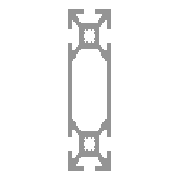
# Autodesk Inventor part: 3 842 992 992-2mm
Saved by Autodesk Inventor 2011 SP1 (Build 150282100, 282)
## iProperties
Created: 2011-02-10
Part Number: 3 842 992 992-2mm
Document SubType Name: Modeling
Designer: S. Wile
Density: 2.71 g/cm^3
Categories: <MemberInstance><Categories><Category DisplayName="Structural Shapes" InternalName="089c4875-fa83-4c05-b084-43b9cc11f5ed" Mnemonic="GRDR"><CategoryParameter DisplayName="Custom Base Point" InternalName="4f1d1b73-316d-484b-a3df-9cbabb16eb77" Mnemonic="shpBasePoint"/><CategoryParameter DisplayName="FG Authored" InternalName="9c666724-f362-4ea7-ac62-f6a007de5c69" Mnemonic="shpFGAuto"/><CategoryParameter DisplayName="Legacy Member ID" InternalName="340afe4f-75d7-48d3-ab7d-943f3c3da468" Mnemonic="LegacyMemberID"/><CategoryParameter DisplayName="Base Length" InternalName="42e34263-8f20-4d0e-ad48-bf1385b87c24" Mnemonic="shplen"/><CategoryParameter DisplayName="Distance of the Center of Gravity X-X" InternalName="26c9bdb8-9c79-4b4f-a92e-8e197583c9c4" Mnemonic="grcendistX"/><CategoryParameter DisplayName="Distance of the Center of Gravity Y-Y" InternalName="bcc4fb17-7af4-436a-8f8c-d0aa3b0248c5" Mnemonic="grcendistY"/><CategoryParameter DisplayName="Torsional Rigidity Modulus" InternalName="26c1ec35-5026-4c63-ad0a-751cf684a536" Mnemonic="torrigmod"/><CategoryParameter DisplayName="Torsional Section Modulus" InternalName="7c55a8dc-8844-49f9-a867-cc677b30ec9a" Mnemonic="torsecmod"/><CategoryParameter DisplayName="Coefficient of Shear Displacement" InternalName="de4c90c6-aaa8-468f-a335-6737b311b5d3" Mnemonic="shdispc"/><CategoryParameter DisplayName="Section Area" InternalName="1ff91680-64b0-4202-b9a3-7fd3f94bba3b" Mnemonic="secarea"/><CategoryParameter DisplayName="Moment of Inertia (x)" InternalName="4cd780bc-73d7-43ac-917a-579e5cbd684d" Mnemonic="inermomx"/><CategoryParameter DisplayName="Moment of Inertia (y)" InternalName="4b9f58ea-bced-460e-81ea-3d29ca5a49e3" Mnemonic="inermomy"/><CategoryParameter DisplayName="Section Module (x)" InternalName="72cfad18-cf51-4ed4-aaa7-c6b224f8419f" Mnemonic="secmodx"/><CategoryParameter DisplayName="Section Module (y)" InternalName="59eaa5e9-d227-48dc-b6c1-6920f96e0f95" Mnemonic="secmody"/><CategoryParameter DisplayName="Radius of Gyration (x)" InternalName="25778675-03e9-40c1-b6a8-4a9ed693320d" Mnemonic="gyrradx"/><CategoryParameter DisplayName="Radius of Gyration (y)" InternalName="bfa18ebe-1636-4dbe-8d42-b263e0b73184" Mnemonic="gyrrady"/><CategoryParameter DisplayName="Shape Thickness" InternalName="d109cf76-8eb4-42fc-9800-4409734adc67" Mnemonic="shpthick"/><CategoryParameter DisplayName="Second Shape Thickness" InternalName="9251a8e1-85fd-4e47-af99-afdb762317d9" Mnemonic="shpthick2"/><CategoryParameter DisplayName="Shape Width" InternalName="7c717d54-a18f-4666-b4d4-573cce22c62c" Mnemonic="shpwdth"/><CategoryParameter DisplayName="Shape Height" InternalName="50274e7d-5ac0-4796-92cb-c59e54983c67" Mnemonic="shpheig"/><CategoryParameter DisplayName="Mass per Length Unit" InternalName="0bb95a10-148f-4027-a459-38d7b056702a" Mnemonic="shpmass"/><CategoryParameter DisplayName="Section Designation" InternalName="5a64d034-428d-49c8-ba32-7619764de20f" Mnemonic="shpdes"/><Category DisplayName="Other" InternalName="f02205ff-2390-476f-921c-0b3185f88e84" Mnemonic="OTHSHP"><CategoryParameter DisplayName="Moment of Inertia (x)" InternalName="ec6737bc-264f-43ed-b0bd-f6d410c2718d" Mnemonic="inermomx"/><CategoryParameter DisplayName="Moment of Inertia (y)" InternalName="044c654e-f649-48ac-84cc-650a29ae31ca" Mnemonic="inermomy"/><CategoryParameter DisplayName="Section Module (x)" InternalName="cac70804-9d39-43bb-be17-56ea1f39a6c2" Mnemonic="secmodx"/><CategoryParameter DisplayName="Section Module (y)" InternalName="88b8bff9-a616-4028-93d5-ed4f79680d13" Mnemonic="secmody"/><CategoryParameter DisplayName="Section Area" InternalName="c46ecdf8-b6eb-4db9-8b25-30258930c1e3" Mnemonic="secarea"/><CategoryParameter DisplayName="Radius of Gyration (x)" InternalName="ee72c61e-565e-4fd6-b448-66e1e1abcb7e" Mnemonic="gyrradx"/><CategoryParameter DisplayName="Radius of Gyration (y)" InternalName="743e1dfe-1bba-408b-b985-cf752b207386" Mnemonic="gyrrady"/><CategoryParameter DisplayName="Shape Thickness" InternalName="12b1a788-9233-48fd-a933-2df8ff42b15f" Mnemonic="shpthick"/><CategoryParameter DisplayName="Mass per Length Unit" InternalName="2fd289d6-9394-4d2d-97e6-6659d7d4551d" Mnemonic="shpmass"/></Category></Category></Categories><FamilyTemplate Id="20x60"><FamilyTemplateParameters><FamilyTemplateParameter ObjectType="kUserParameterObject" ValueType="xs:double" Id="1" ObjectReferenceKey="G_L"/><FamilyTemplateParameter ObjectType="kUserParameterObject" ValueType="xs:double" Id="2" ObjectReferenceKey="G_OFFSET_END"/><FamilyTemplateParameter ObjectType="kUserParameterObject" ValueType="xs:double" Id="3" ObjectReferenceKey="G_OFFSET_START"/><FamilyTemplateParameter ObjectType="kUserParameterObject" ValueType="xs:double" Id="4" ObjectReferenceKey="Length"/><FamilyTemplateParameter ObjectType="kPropertyObject" ValueType="xs:string" Id="7" ObjectReferenceKey="{32853F0F-3444-11d1-9E93-0060B03C1CA6}" SubObjectId="52"/><FamilyTemplateParameter ObjectType="kPartComponentDefinitionObject" ValueType="xs:string" Id="8" SubObjectId="Material"/><FamilyTemplateParameter ObjectType="kPropertyObject" ValueType="xs:string" Id="9" ObjectReferenceKey="{32853F0F-3444-11d1-9E93-0060B03C1CA6}" SubObjectId="5"/><FamilyTemplateParameter ObjectType="kPropertyObject" ValueType="xs:string" Id="10" ObjectReferenceKey="{32853F0F-3444-11D1-9E93-0060B03C1CA6}" SubObjectId="55"/><FamilyTemplateParameter ObjectType="kiPartTableColumnObject" ValueType="xs:string" Id="21" ObjectReferenceKey="FILENAME"/><FamilyTemplateParameter ObjectType="kiPartTableColumnObject" ValueType="xs:string" Id="22" ObjectReferenceKey="MEMBER_REVISION"/></FamilyTemplateParameters></FamilyTemplate><CategoryParameterMap><ParamToTemplateMap><ParamToTemplate CategoryParameter="//CategoryParameter[@InternalName='4f1d1b73-316d-484b-a3df-9cbabb16eb77']" ConstantValue="1"/><ParamToTemplate CategoryParameter="//CategoryParameter[@InternalName='9c666724-f362-4ea7-ac62-f6a007de5c69']" ConstantValue="1"/><ParamToTemplate CategoryParameter="//CategoryParameter[@InternalName='2675968c-4ce5-49e0-a4f5-552d29089031']" TemplateParameter="7"/><ParamToTemplate CategoryParameter="//CategoryParameter[@InternalName='8b46a4cc-9585-4fed-90c3-899f57e09a73']" TemplateParameter="21"/><ParamToTemplate CategoryParameter="//CategoryParameter[@InternalName='42e34263-8f20-4d0e-ad48-bf1385b87c24']" TemplateParameter="4"/><ParamToTemplate CategoryParameter="//CategoryParameter[@InternalName='818a152a-d3c3-49ca-80ee-df7d91421b8e']" TemplateParameter="8"/><ParamToTemplate CategoryParameter="//CategoryParameter[@InternalName='a65d44b9-392f-4f4f-857b-e4b3d54996fe']" TemplateParameter="22"/><ParamToTemplate CategoryParameter="//CategoryParameter[@InternalName='016b6077-bfbe-49bd-92c9-d8d59c39c941']" TemplateParameter="9"/></ParamToTemplateMap></CategoryParameterMap></MemberInstance>
Stock Number: 3 842 992 992
Description: PROFILE 20x60, -/-
Material: Aluminum-6061
Mass: 1.9466 g
Surface Area: 15.1922 cm^2
Volume: 0.718302 cm^3
Author: S. Wile
Autodesk Inventor part; units mm, degrees
ref_plane "YZ Plane" through (0, 0, 0) normal (1, 0, 0) x (0, 1, 0)
ref_plane "XZ Plane" through (0, 0, 0) normal (0, 1, 0) x (-1, 0, 0)
ref_plane "XY Plane" through (0, 0, 0) normal (0, 0, 1) x (1, 0, 0)
sketch "20x60" plane through (0, 0, 0) normal (0, 0, 1) x (1, 0, 0)
  arc A0 (206.0307, 110.0668) -> (206.0307, 112.5831) centre (203.5854, 111.3249) ccw
  line L0 (206.0307, 112.5831) -> (206.5331, 113.212)
  arc A1 (206.5331, 113.212) -> (205.4725, 114.2727) centre (203.5854, 111.3249) ccw
  line L1 (205.4725, 114.2727) -> (204.8436, 113.7702)
  arc A2 (204.8436, 113.7702) -> (202.3272, 113.7702) centre (203.5854, 111.3249) ccw
  line L2 (202.3272, 113.7702) -> (201.6984, 114.2727)
  arc A3 (201.6984, 114.2727) -> (200.6377, 113.212) centre (203.5854, 111.3249) ccw
  line L3 (200.6377, 113.212) -> (201.1401, 112.5831)
  arc A4 (201.1401, 112.5831) -> (201.1401, 110.0668) centre (203.5854, 111.3249) ccw
  line L4 (201.1401, 110.0668) -> (200.6377, 109.4379)
  arc A5 (200.6377, 109.4379) -> (201.6984, 108.3772) centre (203.5854, 111.3249) ccw
  line L5 (201.6984, 108.3772) -> (202.3272, 108.8796)
  arc A6 (202.3272, 108.8796) -> (204.8436, 108.8796) centre (203.5854, 111.3249) ccw
  line L6 (204.8436, 108.8796) -> (205.4725, 108.3772)
  arc A7 (205.4725, 108.3772) -> (206.5331, 109.4379) centre (203.5854, 111.3249) ccw
  line L7 (206.5331, 109.4379) -> (206.0307, 110.0668)
  line L8 (195.0854, 80.8798) -> (199.9996, 75.9656)
  line L9 (197.5854, 63.3192) -> (197.5854, 64.0514)
  arc A8 (197.5854, 63.3192) -> (198.0854, 62.8192) centre (198.0854, 63.3192) ccw
  line L10 (200.0854, 62.8192) -> (198.0854, 62.8192)
  arc A9 (200.5854, 62.3192) -> (200.0854, 62.8192) centre (200.0854, 62.3192) ccw
  line L11 (200.5854, 62.0192) -> (200.5854, 62.3192)
  arc A10 (200.3854, 61.8192) -> (200.5854, 62.0192) centre (200.3854, 62.0192) ccw
  line L12 (200.2354, 61.8192) -> (200.3854, 61.8192)
  arc A11 (200.2354, 61.8192) -> (200.0354, 61.6192) centre (200.2354, 61.6192) ccw
  line L13 (200.0354, 61.5192) -> (200.0354, 61.6192)
  arc A12 (199.8354, 61.3192) -> (200.0354, 61.5192) centre (199.8354, 61.5192) ccw
  line L14 (195.0854, 61.3192) -> (199.8354, 61.3192)
  arc A13 (193.5854, 62.8192) -> (195.0854, 61.3192) centre (195.0854, 62.8192) ccw
  line L15 (193.5854, 67.5692) -> (193.5854, 62.8192)
  arc A14 (193.7854, 67.7692) -> (193.5854, 67.5692) centre (193.7854, 67.5692) ccw
  line L16 (193.8854, 67.7692) -> (193.7854, 67.7692)
  arc A15 (193.8854, 67.7692) -> (194.0854, 67.9692) centre (193.8854, 67.9692) ccw
  line L17 (194.0854, 68.1192) -> (194.0854, 67.9692)
  arc A16 (194.2854, 68.3192) -> (194.0854, 68.1192) centre (194.2854, 68.1192) ccw
  line L18 (194.5854, 68.3192) -> (194.2854, 68.3192)
  arc A17 (195.0854, 67.8192) -> (194.5854, 68.3192) centre (194.5854, 67.8192) ccw
  line L19 (195.0854, 65.8192) -> (195.0854, 67.8192)
  arc A18 (195.0854, 65.8192) -> (195.5854, 65.3192) centre (195.5854, 65.8192) ccw
  line L20 (196.1177, 65.3192) -> (195.5854, 65.3192)
  arc A19 (196.1177, 65.3192) -> (196.4712, 65.4656) centre (196.1177, 65.8192) ccw
  line L21 (198.864, 67.8584) -> (196.4712, 65.4656)
  arc A20 (198.864, 67.8584) -> (199.0104, 68.2119) centre (198.5104, 68.2119) ccw
  line L22 (199.0104, 70.2357) -> (199.0104, 68.2119)
  arc A21 (199.0372, 70.3357) -> (199.0104, 70.2357) centre (199.2104, 70.2357) ccw
  line L23 (199.5473, 71.2192) -> (199.0372, 70.3357)
  arc A22 (199.5473, 71.2192) -> (199.5473, 71.4192) centre (199.3741, 71.3192) ccw
  line L24 (199.0372, 72.3027) -> (199.5473, 71.4192)
  arc A23 (199.0104, 72.4027) -> (199.0372, 72.3027) centre (199.2104, 72.4027) ccw
  line L25 (199.0104, 74.4264) -> (199.0104, 72.4027)
  arc A24 (199.0104, 74.4264) -> (198.864, 74.7799) centre (198.5104, 74.4264) ccw
  line L26 (196.4712, 77.1727) -> (198.864, 74.7799)
  arc A25 (196.4712, 77.1727) -> (196.1177, 77.3192) centre (196.1177, 76.8192) ccw
  line L27 (195.5854, 77.3192) -> (196.1177, 77.3192)
  arc A26 (195.5854, 77.3192) -> (195.0854, 76.8192) centre (195.5854, 76.8192) ccw
  line L28 (195.0854, 74.8192) -> (195.0854, 76.8192)
  arc A27 (194.5854, 74.3192) -> (195.0854, 74.8192) centre (194.5854, 74.8192) ccw
  line L29 (194.2854, 74.3192) -> (194.5854, 74.3192)
  arc A28 (194.0854, 74.5192) -> (194.2854, 74.3192) centre (194.2854, 74.5192) ccw
  line L30 (194.0854, 74.6692) -> (194.0854, 74.5192)
  arc A29 (194.0854, 74.6692) -> (193.8854, 74.8692) centre (193.8854, 74.6692) ccw
  line L31 (193.7854, 74.8692) -> (193.8854, 74.8692)
  arc A30 (193.5854, 75.0692) -> (193.7854, 74.8692) centre (193.7854, 75.0692) ccw
  line L32 (193.5854, 107.5749) -> (193.5854, 75.0692)
  arc A31 (204.8436, 73.7645) -> (202.3231, 73.7623) centre (203.5854, 71.3192) ccw
  line L33 (202.3231, 73.7623) -> (201.6715, 74.3088)
  arc A32 (201.6715, 74.3088) -> (200.5932, 73.2291) centre (203.5854, 71.3192) ccw
  line L34 (200.5932, 73.2291) -> (201.1401, 72.5773)
  arc A33 (201.1401, 72.5773) -> (201.1423, 70.0568) centre (203.5854, 71.3192) ccw
  line L35 (201.1423, 70.0568) -> (200.5958, 69.4053)
  arc A34 (200.5958, 69.4053) -> (201.6755, 68.327) centre (203.5854, 71.3192) ccw
  line L36 (201.6755, 68.327) -> (202.3272, 68.8739)
  arc A35 (202.3272, 68.8739) -> (204.8478, 68.876) centre (203.5854, 71.3192) ccw
  line L37 (204.8478, 68.876) -> (205.4993, 68.3295)
  arc A36 (205.4993, 68.3295) -> (206.5776, 69.4092) centre (203.5854, 71.3192) ccw
  line L38 (206.5776, 69.4092) -> (206.0307, 70.061)
  arc A37 (206.0307, 70.061) -> (206.0307, 72.5773) centre (203.5854, 71.3192) ccw
  line L39 (206.0307, 72.5773) -> (206.5751, 73.2331)
  arc A38 (206.5751, 73.2331) -> (205.4954, 74.3113) centre (203.5854, 71.3192) ccw
  line L40 (205.4954, 74.3113) -> (204.8436, 73.7645)
  line L41 (213.5854, 114.9749) -> (213.5854, 119.8192)
  arc A39 (213.3854, 114.7749) -> (213.5854, 114.9749) centre (213.3854, 114.9749) ccw
  line L42 (213.2854, 114.7749) -> (213.3854, 114.7749)
  arc A40 (213.2854, 114.7749) -> (213.0854, 114.5749) centre (213.2854, 114.5749) ccw
  line L43 (213.0854, 114.4749) -> (213.0854, 114.5749)
  arc A41 (212.8854, 114.2749) -> (213.0854, 114.4749) centre (212.8854, 114.4749) ccw
  line L44 (212.5854, 114.2749) -> (212.8854, 114.2749)
  arc A42 (212.0854, 114.7749) -> (212.5854, 114.2749) centre (212.5854, 114.7749) ccw
  line L45 (212.0854, 116.8249) -> (212.0854, 114.7749)
  arc A43 (212.0854, 116.8249) -> (211.5854, 117.3249) centre (211.5854, 116.8249) ccw
  line L46 (210.8532, 117.3249) -> (211.5854, 117.3249)
  arc A44 (210.8532, 117.3249) -> (210.4996, 117.1785) centre (210.8532, 116.8249) ccw
  line L47 (208.3069, 114.9857) -> (210.4996, 117.1785)
  arc A45 (208.3069, 114.9857) -> (208.1604, 114.6322) centre (208.6604, 114.6322) ccw
  line L48 (208.1604, 112.3035) -> (208.1604, 114.6322)
  arc A46 (208.1336, 112.2035) -> (208.1604, 112.3035) centre (207.9604, 112.3035) ccw
  line L49 (207.7274, 111.4999) -> (208.1336, 112.2035)
  arc A47 (207.7274, 111.4999) -> (207.7274, 111.2999) centre (207.9006, 111.3999) ccw
  line L50 (208.1336, 110.5964) -> (207.7274, 111.2999)
  arc A48 (208.1604, 110.4964) -> (208.1336, 110.5964) centre (207.9604, 110.4964) ccw
  line L51 (208.1604, 108.0177) -> (208.1604, 110.4964)
  arc A49 (208.1604, 108.0177) -> (208.3069, 107.6642) centre (208.6604, 108.0177) ccw
  line L52 (210.4996, 105.4714) -> (208.3069, 107.6642)
  arc A50 (210.4996, 105.4714) -> (210.8532, 105.3249) centre (210.8532, 105.8249) ccw
  line L53 (211.5854, 105.3249) -> (210.8532, 105.3249)
  arc A51 (211.5854, 105.3249) -> (212.0854, 105.8249) centre (211.5854, 105.8249) ccw
  line L54 (212.0854, 107.7749) -> (212.0854, 105.8249)
  arc A52 (212.5854, 108.2749) -> (212.0854, 107.7749) centre (212.5854, 107.7749) ccw
  line L55 (212.8854, 108.2749) -> (212.5854, 108.2749)
  arc A53 (213.0854, 108.0749) -> (212.8854, 108.2749) centre (212.8854, 108.0749) ccw
  line L56 (213.0854, 107.9749) -> (213.0854, 108.0749)
  arc A54 (213.0854, 107.9749) -> (213.2854, 107.7749) centre (213.2854, 107.9749) ccw
  line L57 (213.3854, 107.7749) -> (213.2854, 107.7749)
  arc A55 (213.5854, 107.5749) -> (213.3854, 107.7749) centre (213.3854, 107.5749) ccw
  line L58 (213.5854, 75.0192) -> (213.5854, 107.5749)
  arc A56 (213.3854, 74.8192) -> (213.5854, 75.0192) centre (213.3854, 75.0192) ccw
  line L59 (213.2854, 74.8192) -> (213.3854, 74.8192)
  arc A57 (213.2854, 74.8192) -> (213.0854, 74.6192) centre (213.2854, 74.6192) ccw
  line L60 (213.0854, 74.5192) -> (213.0854, 74.6192)
  arc A58 (212.8854, 74.3192) -> (213.0854, 74.5192) centre (212.8854, 74.5192) ccw
  line L61 (212.5854, 74.3192) -> (212.8854, 74.3192)
  arc A59 (212.0854, 74.8192) -> (212.5854, 74.3192) centre (212.5854, 74.8192) ccw
  line L62 (212.0854, 76.8192) -> (212.0854, 74.8192)
  arc A60 (212.0854, 76.8192) -> (211.5854, 77.3192) centre (211.5854, 76.8192) ccw
  line L63 (211.0532, 77.3192) -> (211.5854, 77.3192)
  arc A61 (211.0532, 77.3192) -> (210.6996, 77.1727) centre (211.0532, 76.8192) ccw
  line L64 (208.3069, 74.7799) -> (210.6996, 77.1727)
  arc A62 (208.3069, 74.7799) -> (208.1604, 74.4264) centre (208.6604, 74.4264) ccw
  line L65 (208.1604, 72.4027) -> (208.1604, 74.4264)
  arc A63 (208.1336, 72.3027) -> (208.1604, 72.4027) centre (207.9604, 72.4027) ccw
  line L66 (207.6235, 71.4192) -> (208.1336, 72.3027)
  arc A64 (207.6235, 71.4192) -> (207.6235, 71.2192) centre (207.7967, 71.3192) ccw
  line L67 (208.1336, 70.3357) -> (207.6235, 71.2192)
  arc A65 (208.1604, 70.2357) -> (208.1336, 70.3357) centre (207.9604, 70.2357) ccw
  line L68 (208.1604, 68.2119) -> (208.1604, 70.2357)
  arc A66 (208.1604, 68.2119) -> (208.3069, 67.8584) centre (208.6604, 68.2119) ccw
  line L69 (210.6996, 65.4656) -> (208.3069, 67.8584)
  arc A67 (210.6996, 65.4656) -> (211.0532, 65.3192) centre (211.0532, 65.8192) ccw
  line L70 (211.5854, 65.3192) -> (211.0532, 65.3192)
  arc A68 (211.5854, 65.3192) -> (212.0854, 65.8192) centre (211.5854, 65.8192) ccw
  line L71 (212.0854, 67.8192) -> (212.0854, 65.8192)
  arc A69 (212.5854, 68.3192) -> (212.0854, 67.8192) centre (212.5854, 67.8192) ccw
  line L72 (212.8854, 68.3192) -> (212.5854, 68.3192)
  arc A70 (213.0854, 68.1192) -> (212.8854, 68.3192) centre (212.8854, 68.1192) ccw
  line L73 (213.0854, 68.0192) -> (213.0854, 68.1192)
  arc A71 (213.0854, 68.0192) -> (213.2854, 67.8192) centre (213.2854, 68.0192) ccw
  line L74 (213.3854, 67.8192) -> (213.2854, 67.8192)
  arc A72 (213.5854, 67.6192) -> (213.3854, 67.8192) centre (213.3854, 67.6192) ccw
  line L75 (213.5854, 62.8192) -> (213.5854, 67.6192)
  arc A73 (212.0854, 61.3192) -> (213.5854, 62.8192) centre (212.0854, 62.8192) ccw
  line L76 (207.3354, 61.3192) -> (212.0854, 61.3192)
  arc A74 (207.1354, 61.5192) -> (207.3354, 61.3192) centre (207.3354, 61.5192) ccw
  line L77 (207.1354, 61.6192) -> (207.1354, 61.5192)
  arc A75 (207.1354, 61.6192) -> (206.9354, 61.8192) centre (206.9354, 61.6192) ccw
  line L78 (206.7854, 61.8192) -> (206.9354, 61.8192)
  arc A76 (206.5854, 62.0192) -> (206.7854, 61.8192) centre (206.7854, 62.0192) ccw
  line L79 (206.5854, 62.3192) -> (206.5854, 62.0192)
  arc A77 (207.0854, 62.8192) -> (206.5854, 62.3192) centre (207.0854, 62.3192) ccw
  line L80 (209.0854, 62.8192) -> (207.0854, 62.8192)
  arc A78 (209.0854, 62.8192) -> (209.5854, 63.3192) centre (209.0854, 63.3192) ccw
  line L81 (209.5854, 64.0514) -> (209.5854, 63.3192)
  arc A79 (209.5854, 64.0514) -> (209.439, 64.4049) centre (209.0854, 64.0514) ccw
  line L82 (207.1712, 66.6727) -> (209.439, 64.4049)
  arc A80 (207.1712, 66.6727) -> (206.8177, 66.8192) centre (206.8177, 66.3192) ccw
  line L83 (204.539, 66.8192) -> (206.8177, 66.8192)
  arc A81 (204.439, 66.846) -> (204.539, 66.8192) centre (204.539, 67.0192) ccw
  line L84 (203.6854, 67.281) -> (204.439, 66.846)
  arc A82 (203.6854, 67.281) -> (203.4854, 67.281) centre (203.5854, 67.1078) ccw
  line L85 (202.7318, 66.846) -> (203.4854, 67.281)
  arc A83 (202.6318, 66.8192) -> (202.7318, 66.846) centre (202.6318, 67.0192) ccw
  line L86 (200.3532, 66.8192) -> (202.6318, 66.8192)
  arc A84 (200.3532, 66.8192) -> (199.9996, 66.6727) centre (200.3532, 66.3192) ccw
  line L87 (197.7319, 64.4049) -> (199.9996, 66.6727)
  arc A85 (197.7319, 64.4049) -> (197.5854, 64.0514) centre (198.0854, 64.0514) ccw
  arc A86 (199.9996, 75.9656) -> (200.3532, 75.8192) centre (200.3532, 76.3192) ccw
  line L88 (200.3532, 75.8192) -> (202.6318, 75.8192)
  arc A87 (202.7318, 75.7924) -> (202.6318, 75.8192) centre (202.6318, 75.6192) ccw
  line L89 (202.7318, 75.7924) -> (203.4854, 75.3573)
  arc A88 (203.4854, 75.3573) -> (203.6854, 75.3573) centre (203.5854, 75.5305) ccw
  line L90 (203.6854, 75.3573) -> (204.439, 75.7924)
  arc A89 (204.539, 75.8192) -> (204.439, 75.7924) centre (204.539, 75.6192) ccw
  line L91 (204.539, 75.8192) -> (206.8177, 75.8192)
  arc A90 (206.8177, 75.8192) -> (207.1712, 75.9656) centre (206.8177, 76.3192) ccw
  line L92 (207.1712, 75.9656) -> (212.0854, 80.8798)
  line L93 (212.0854, 80.8798) -> (212.0854, 101.7643)
  line L94 (212.0854, 101.7643) -> (207.1712, 106.6785)
  arc A91 (207.1712, 106.6785) -> (206.8177, 106.8249) centre (206.8177, 106.3249) ccw
  line L95 (206.8177, 106.8249) -> (204.539, 106.8249)
  arc A92 (204.439, 106.8517) -> (204.539, 106.8249) centre (204.539, 107.0249) ccw
  line L96 (204.439, 106.8517) -> (203.6854, 107.2868)
  arc A93 (203.6854, 107.2868) -> (203.4854, 107.2868) centre (203.5854, 107.1136) ccw
  line L97 (203.4854, 107.2868) -> (202.7318, 106.8517)
  arc A94 (202.6318, 106.8249) -> (202.7318, 106.8517) centre (202.6318, 107.0249) ccw
  line L98 (202.6318, 106.8249) -> (200.3532, 106.8249)
  arc A95 (200.3532, 106.8249) -> (199.9996, 106.6785) centre (200.3532, 106.3249) ccw
  line L99 (199.9996, 106.6785) -> (195.0854, 101.7643)
  line L100 (195.0854, 101.7643) -> (195.0854, 80.8798)
  arc A96 (193.7854, 107.7749) -> (193.5854, 107.5749) centre (193.7854, 107.5749) ccw
  line L101 (193.8854, 107.7749) -> (193.7854, 107.7749)
  arc A97 (193.8854, 107.7749) -> (194.0854, 107.9749) centre (193.8854, 107.9749) ccw
  line L102 (194.0854, 108.0749) -> (194.0854, 107.9749)
  arc A98 (194.2854, 108.2749) -> (194.0854, 108.0749) centre (194.2854, 108.0749) ccw
  line L103 (194.5854, 108.2749) -> (194.2854, 108.2749)
  arc A99 (195.0854, 107.7749) -> (194.5854, 108.2749) centre (194.5854, 107.7749) ccw
  line L104 (195.0854, 105.8249) -> (195.0854, 107.7749)
  arc A100 (195.0854, 105.8249) -> (195.5854, 105.3249) centre (195.5854, 105.8249) ccw
  line L105 (196.3177, 105.3249) -> (195.5854, 105.3249)
  arc A101 (196.3177, 105.3249) -> (196.6712, 105.4714) centre (196.3177, 105.8249) ccw
  line L106 (198.864, 107.6642) -> (196.6712, 105.4714)
  arc A102 (198.864, 107.6642) -> (199.0104, 108.0177) centre (198.5104, 108.0177) ccw
  line L107 (199.0104, 110.4964) -> (199.0104, 108.0177)
  arc A103 (199.0372, 110.5964) -> (199.0104, 110.4964) centre (199.2104, 110.4964) ccw
  line L108 (199.4434, 111.2999) -> (199.0372, 110.5964)
  arc A104 (199.4434, 111.2999) -> (199.4434, 111.4999) centre (199.2702, 111.3999) ccw
  line L109 (199.0372, 112.2035) -> (199.4434, 111.4999)
  arc A105 (199.0104, 112.3035) -> (199.0372, 112.2035) centre (199.2104, 112.3035) ccw
  line L110 (199.0104, 114.6322) -> (199.0104, 112.3035)
  arc A106 (199.0104, 114.6322) -> (198.864, 114.9857) centre (198.5104, 114.6322) ccw
  line L111 (196.6712, 117.1785) -> (198.864, 114.9857)
  arc A107 (196.6712, 117.1785) -> (196.3177, 117.3249) centre (196.3177, 116.8249) ccw
  line L112 (195.5854, 117.3249) -> (196.3177, 117.3249)
  arc A108 (195.5854, 117.3249) -> (195.0854, 116.8249) centre (195.5854, 116.8249) ccw
  line L113 (195.0854, 114.7749) -> (195.0854, 116.8249)
  arc A109 (194.5854, 114.2749) -> (195.0854, 114.7749) centre (194.5854, 114.7749) ccw
  line L114 (194.2854, 114.2749) -> (194.5854, 114.2749)
  arc A110 (194.0854, 114.4749) -> (194.2854, 114.2749) centre (194.2854, 114.4749) ccw
  line L115 (194.0854, 114.5749) -> (194.0854, 114.4749)
  arc A111 (194.0854, 114.5749) -> (193.8854, 114.7749) centre (193.8854, 114.5749) ccw
  line L116 (193.7854, 114.7749) -> (193.8854, 114.7749)
  arc A112 (193.5854, 114.9749) -> (193.7854, 114.7749) centre (193.7854, 114.9749) ccw
  line L117 (193.5854, 119.8192) -> (193.5854, 114.9749)
  arc A113 (195.0854, 121.3192) -> (193.5854, 119.8192) centre (195.0854, 119.8192) ccw
  line L118 (199.8354, 121.3192) -> (195.0854, 121.3192)
  arc A114 (200.0354, 121.1192) -> (199.8354, 121.3192) centre (199.8354, 121.1192) ccw
  line L119 (200.0354, 121.0192) -> (200.0354, 121.1192)
  arc A115 (200.0354, 121.0192) -> (200.2354, 120.8192) centre (200.2354, 121.0192) ccw
  line L120 (200.3854, 120.8192) -> (200.2354, 120.8192)
  arc A116 (200.5854, 120.6192) -> (200.3854, 120.8192) centre (200.3854, 120.6192) ccw
  line L121 (200.5854, 120.3192) -> (200.5854, 120.6192)
  arc A117 (200.0854, 119.8192) -> (200.5854, 120.3192) centre (200.0854, 120.3192) ccw
  line L122 (198.0854, 119.8192) -> (200.0854, 119.8192)
  arc A118 (198.0854, 119.8192) -> (197.5854, 119.3192) centre (198.0854, 119.3192) ccw
  line L123 (197.5854, 118.5869) -> (197.5854, 119.3192)
  arc A119 (197.5854, 118.5869) -> (197.7319, 118.2334) centre (198.0854, 118.5869) ccw
  line L124 (199.9996, 115.9656) -> (197.7319, 118.2334)
  arc A120 (199.9996, 115.9656) -> (200.3532, 115.8192) centre (200.3532, 116.3192) ccw
  line L125 (202.6318, 115.8192) -> (200.3532, 115.8192)
  arc A121 (202.7318, 115.7924) -> (202.6318, 115.8192) centre (202.6318, 115.6192) ccw
  line L126 (203.5262, 115.3337) -> (202.7318, 115.7924)
  arc A122 (203.5262, 115.3337) -> (203.6446, 115.3337) centre (203.5854, 115.4363) ccw
  line L127 (204.439, 115.7924) -> (203.6446, 115.3337)
  arc A123 (204.539, 115.8192) -> (204.439, 115.7924) centre (204.539, 115.6192) ccw
  line L128 (206.8177, 115.8192) -> (204.539, 115.8192)
  arc A124 (206.8177, 115.8192) -> (207.1712, 115.9656) centre (206.8177, 116.3192) ccw
  line L129 (209.439, 118.2334) -> (207.1712, 115.9656)
  arc A125 (209.439, 118.2334) -> (209.5854, 118.5869) centre (209.0854, 118.5869) ccw
  line L130 (209.5854, 119.3192) -> (209.5854, 118.5869)
  arc A126 (209.5854, 119.3192) -> (209.0854, 119.8192) centre (209.0854, 119.3192) ccw
  line L131 (207.0854, 119.8192) -> (209.0854, 119.8192)
  arc A127 (206.5854, 120.3192) -> (207.0854, 119.8192) centre (207.0854, 120.3192) ccw
  line L132 (206.5854, 120.6192) -> (206.5854, 120.3192)
  arc A128 (206.7854, 120.8192) -> (206.5854, 120.6192) centre (206.7854, 120.6192) ccw
  line L133 (206.9354, 120.8192) -> (206.7854, 120.8192)
  arc A129 (206.9354, 120.8192) -> (207.1354, 121.0192) centre (206.9354, 121.0192) ccw
  line L134 (207.1354, 121.1192) -> (207.1354, 121.0192)
  arc A130 (207.3354, 121.3192) -> (207.1354, 121.1192) centre (207.3354, 121.1192) ccw
  line L135 (212.0854, 121.3192) -> (207.3354, 121.3192)
  arc A131 (213.5854, 119.8192) -> (212.0854, 121.3192) centre (212.0854, 119.8192) ccw
sketch "Sketch1" plane through (0, 0, 0) normal (0, 0, 1) x (1, 0, 0)
  arc A0 (2.4453, -1.2582) -> (2.4453, 1.2582) centre (0, 0) ccw
  line L0 (2.4453, 1.2582) -> (2.9477, 1.8871)
  arc A1 (2.9477, 1.8871) -> (1.8871, 2.9477) centre (0, 0) ccw
  line L1 (1.8871, 2.9477) -> (1.2582, 2.4453)
  arc A2 (1.2582, 2.4453) -> (-1.2582, 2.4453) centre (0, 0) ccw
  line L2 (-1.2582, 2.4453) -> (-1.8871, 2.9477)
  arc A3 (-1.8871, 2.9477) -> (-2.9477, 1.8871) centre (0, 0) ccw
  line L3 (-2.9477, 1.8871) -> (-2.4453, 1.2582)
  arc A4 (-2.4453, 1.2582) -> (-2.4453, -1.2582) centre (0, 0) ccw
  line L4 (-2.4453, -1.2582) -> (-2.9477, -1.8871)
  arc A5 (-2.9477, -1.8871) -> (-1.8871, -2.9477) centre (0, 0) ccw
  line L5 (-1.8871, -2.9477) -> (-1.2582, -2.4453)
  arc A6 (-1.2582, -2.4453) -> (1.2582, -2.4453) centre (0, 0) ccw
  line L6 (1.2582, -2.4453) -> (1.8871, -2.9477)
  arc A7 (1.8871, -2.9477) -> (2.9477, -1.8871) centre (0, 0) ccw
  line L7 (2.9477, -1.8871) -> (2.4453, -1.2582)
  line L8 (-8.5, -30.4451) -> (-3.5858, -35.3593)
  line L9 (-6, -48.0058) -> (-6, -47.2735)
  arc A8 (-6, -48.0058) -> (-5.5, -48.5058) centre (-5.5, -48.0058) ccw
  line L10 (-3.5, -48.5058) -> (-5.5, -48.5058)
  arc A9 (-3, -49.0058) -> (-3.5, -48.5058) centre (-3.5, -49.0058) ccw
  line L11 (-3, -49.3058) -> (-3, -49.0058)
  arc A10 (-3.2, -49.5058) -> (-3, -49.3058) centre (-3.2, -49.3058) ccw
  line L12 (-3.35, -49.5058) -> (-3.2, -49.5058)
  arc A11 (-3.35, -49.5058) -> (-3.55, -49.7058) centre (-3.35, -49.7058) ccw
  line L13 (-3.55, -49.8058) -> (-3.55, -49.7058)
  arc A12 (-3.75, -50.0058) -> (-3.55, -49.8058) centre (-3.75, -49.8058) ccw
  line L14 (-8.5, -50.0058) -> (-3.75, -50.0058)
  arc A13 (-10, -48.5058) -> (-8.5, -50.0058) centre (-8.5, -48.5058) ccw
  line L15 (-10, -43.7558) -> (-10, -48.5058)
  arc A14 (-9.8, -43.5558) -> (-10, -43.7558) centre (-9.8, -43.7558) ccw
  line L16 (-9.7, -43.5558) -> (-9.8, -43.5558)
  arc A15 (-9.7, -43.5558) -> (-9.5, -43.3558) centre (-9.7, -43.3558) ccw
  line L17 (-9.5, -43.2058) -> (-9.5, -43.3558)
  arc A16 (-9.3, -43.0058) -> (-9.5, -43.2058) centre (-9.3, -43.2058) ccw
  line L18 (-9, -43.0058) -> (-9.3, -43.0058)
  arc A17 (-8.5, -43.5058) -> (-9, -43.0058) centre (-9, -43.5058) ccw
  line L19 (-8.5, -45.5058) -> (-8.5, -43.5058)
  arc A18 (-8.5, -45.5058) -> (-8, -46.0058) centre (-8, -45.5058) ccw
  line L20 (-7.4678, -46.0058) -> (-8, -46.0058)
  arc A19 (-7.4678, -46.0058) -> (-7.1142, -45.8593) centre (-7.4678, -45.5058) ccw
  line L21 (-4.7214, -43.4666) -> (-7.1142, -45.8593)
  arc A20 (-4.7214, -43.4666) -> (-4.575, -43.113) centre (-5.075, -43.113) ccw
  line L22 (-4.575, -41.0893) -> (-4.575, -43.113)
  arc A21 (-4.5482, -40.9893) -> (-4.575, -41.0893) centre (-4.375, -41.0893) ccw
  line L23 (-4.0381, -40.1058) -> (-4.5482, -40.9893)
  arc A22 (-4.0381, -40.1058) -> (-4.0381, -39.9058) centre (-4.2113, -40.0058) ccw
  line L24 (-4.5482, -39.0223) -> (-4.0381, -39.9058)
  arc A23 (-4.575, -38.9223) -> (-4.5482, -39.0223) centre (-4.375, -38.9223) ccw
  line L25 (-4.575, -36.8985) -> (-4.575, -38.9223)
  arc A24 (-4.575, -36.8985) -> (-4.7214, -36.545) centre (-5.075, -36.8985) ccw
  line L26 (-7.1142, -34.1522) -> (-4.7214, -36.545)
  arc A25 (-7.1142, -34.1522) -> (-7.4678, -34.0058) centre (-7.4678, -34.5058) ccw
  line L27 (-8, -34.0058) -> (-7.4678, -34.0058)
  arc A26 (-8, -34.0058) -> (-8.5, -34.5058) centre (-8, -34.5058) ccw
  line L28 (-8.5, -36.5058) -> (-8.5, -34.5058)
  arc A27 (-9, -37.0058) -> (-8.5, -36.5058) centre (-9, -36.5058) ccw
  line L29 (-9.3, -37.0058) -> (-9, -37.0058)
  arc A28 (-9.5, -36.8058) -> (-9.3, -37.0058) centre (-9.3, -36.8058) ccw
  line L30 (-9.5, -36.6558) -> (-9.5, -36.8058)
  arc A29 (-9.5, -36.6558) -> (-9.7, -36.4558) centre (-9.7, -36.6558) ccw
  line L31 (-9.8, -36.4558) -> (-9.7, -36.4558)
  arc A30 (-10, -36.2558) -> (-9.8, -36.4558) centre (-9.8, -36.2558) ccw
  line L32 (-10, -3.75) -> (-10, -36.2558)
  arc A31 (1.2582, -37.5605) -> (-1.2623, -37.5626) centre (0, -40.0058) ccw
  line L33 (-1.2623, -37.5626) -> (-1.9139, -37.0161)
  arc A32 (-1.9139, -37.0161) -> (-2.9922, -38.0959) centre (0, -40.0058) ccw
  line L34 (-2.9922, -38.0959) -> (-2.4453, -38.7476)
  arc A33 (-2.4453, -38.7476) -> (-2.4431, -41.2681) centre (0, -40.0058) ccw
  line L35 (-2.4431, -41.2681) -> (-2.9897, -41.9196)
  arc A34 (-2.9897, -41.9196) -> (-1.9099, -42.998) centre (0, -40.0058) ccw
  line L36 (-1.9099, -42.998) -> (-1.2582, -42.4511)
  arc A35 (-1.2582, -42.4511) -> (1.2623, -42.4489) centre (0, -40.0058) ccw
  line L37 (1.2623, -42.4489) -> (1.9139, -42.9954)
  arc A36 (1.9139, -42.9954) -> (2.9922, -41.9157) centre (0, -40.0058) ccw
  line L38 (2.9922, -41.9157) -> (2.4453, -41.264)
  arc A37 (2.4453, -41.264) -> (2.4453, -38.7476) centre (0, -40.0058) ccw
  line L39 (2.4453, -38.7476) -> (2.9896, -38.0919)
  arc A38 (2.9896, -38.0919) -> (1.9099, -37.0136) centre (0, -40.0058) ccw
  line L40 (1.9099, -37.0136) -> (1.2582, -37.5605)
  line L41 (10, 3.65) -> (10, 8.4942)
  arc A39 (9.8, 3.45) -> (10, 3.65) centre (9.8, 3.65) ccw
  line L42 (9.7, 3.45) -> (9.8, 3.45)
  arc A40 (9.7, 3.45) -> (9.5, 3.25) centre (9.7, 3.25) ccw
  line L43 (9.5, 3.15) -> (9.5, 3.25)
  arc A41 (9.3, 2.95) -> (9.5, 3.15) centre (9.3, 3.15) ccw
  line L44 (9, 2.95) -> (9.3, 2.95)
  arc A42 (8.5, 3.45) -> (9, 2.95) centre (9, 3.45) ccw
  line L45 (8.5, 5.5) -> (8.5, 3.45)
  arc A43 (8.5, 5.5) -> (8, 6) centre (8, 5.5) ccw
  line L46 (7.2678, 6) -> (8, 6)
  arc A44 (7.2678, 6) -> (6.9142, 5.8536) centre (7.2678, 5.5) ccw
  line L47 (4.7214, 3.6608) -> (6.9142, 5.8536)
  arc A45 (4.7214, 3.6608) -> (4.575, 3.3072) centre (5.075, 3.3072) ccw
  line L48 (4.575, 0.9786) -> (4.575, 3.3072)
  arc A46 (4.5482, 0.8786) -> (4.575, 0.9786) centre (4.375, 0.9786) ccw
  line L49 (4.142, 0.175) -> (4.5482, 0.8786)
  arc A47 (4.142, 0.175) -> (4.142, -0.025) centre (4.3152, 0.075) ccw
  line L50 (4.5482, -0.7286) -> (4.142, -0.025)
  arc A48 (4.575, -0.8286) -> (4.5482, -0.7286) centre (4.375, -0.8286) ccw
  line L51 (4.575, -3.3072) -> (4.575, -0.8286)
  arc A49 (4.575, -3.3072) -> (4.7214, -3.6608) centre (5.075, -3.3072) ccw
  line L52 (6.9142, -5.8536) -> (4.7214, -3.6608)
  arc A50 (6.9142, -5.8536) -> (7.2678, -6) centre (7.2678, -5.5) ccw
  line L53 (8, -6) -> (7.2678, -6)
  arc A51 (8, -6) -> (8.5, -5.5) centre (8, -5.5) ccw
  line L54 (8.5, -3.55) -> (8.5, -5.5)
  arc A52 (9, -3.05) -> (8.5, -3.55) centre (9, -3.55) ccw
  line L55 (9.3, -3.05) -> (9, -3.05)
  arc A53 (9.5, -3.25) -> (9.3, -3.05) centre (9.3, -3.25) ccw
  line L56 (9.5, -3.35) -> (9.5, -3.25)
  arc A54 (9.5, -3.35) -> (9.7, -3.55) centre (9.7, -3.35) ccw
  line L57 (9.8, -3.55) -> (9.7, -3.55)
  arc A55 (10, -3.75) -> (9.8, -3.55) centre (9.8, -3.75) ccw
  line L58 (10, -36.3058) -> (10, -3.75)
  arc A56 (9.8, -36.5058) -> (10, -36.3058) centre (9.8, -36.3058) ccw
  line L59 (9.7, -36.5058) -> (9.8, -36.5058)
  arc A57 (9.7, -36.5058) -> (9.5, -36.7058) centre (9.7, -36.7058) ccw
  line L60 (9.5, -36.8058) -> (9.5, -36.7058)
  arc A58 (9.3, -37.0058) -> (9.5, -36.8058) centre (9.3, -36.8058) ccw
  line L61 (9, -37.0058) -> (9.3, -37.0058)
  arc A59 (8.5, -36.5058) -> (9, -37.0058) centre (9, -36.5058) ccw
  line L62 (8.5, -34.5058) -> (8.5, -36.5058)
  arc A60 (8.5, -34.5058) -> (8, -34.0058) centre (8, -34.5058) ccw
  line L63 (7.4678, -34.0058) -> (8, -34.0058)
  arc A61 (7.4678, -34.0058) -> (7.1142, -34.1522) centre (7.4678, -34.5058) ccw
  line L64 (4.7214, -36.545) -> (7.1142, -34.1522)
  arc A62 (4.7214, -36.545) -> (4.575, -36.8985) centre (5.075, -36.8985) ccw
  line L65 (4.575, -38.9223) -> (4.575, -36.8985)
  arc A63 (4.5482, -39.0223) -> (4.575, -38.9223) centre (4.375, -38.9223) ccw
  line L66 (4.0381, -39.9058) -> (4.5482, -39.0223)
  arc A64 (4.0381, -39.9058) -> (4.0381, -40.1058) centre (4.2113, -40.0058) ccw
  line L67 (4.5482, -40.9893) -> (4.0381, -40.1058)
  arc A65 (4.575, -41.0893) -> (4.5482, -40.9893) centre (4.375, -41.0893) ccw
  line L68 (4.575, -43.113) -> (4.575, -41.0893)
  arc A66 (4.575, -43.113) -> (4.7214, -43.4666) centre (5.075, -43.113) ccw
  line L69 (7.1142, -45.8593) -> (4.7214, -43.4666)
  arc A67 (7.1142, -45.8593) -> (7.4678, -46.0058) centre (7.4678, -45.5058) ccw
  line L70 (8, -46.0058) -> (7.4678, -46.0058)
  arc A68 (8, -46.0058) -> (8.5, -45.5058) centre (8, -45.5058) ccw
  line L71 (8.5, -43.5058) -> (8.5, -45.5058)
  arc A69 (9, -43.0058) -> (8.5, -43.5058) centre (9, -43.5058) ccw
  line L72 (9.3, -43.0058) -> (9, -43.0058)
  arc A70 (9.5, -43.2058) -> (9.3, -43.0058) centre (9.3, -43.2058) ccw
  line L73 (9.5, -43.3058) -> (9.5, -43.2058)
  arc A71 (9.5, -43.3058) -> (9.7, -43.5058) centre (9.7, -43.3058) ccw
  line L74 (9.8, -43.5058) -> (9.7, -43.5058)
  arc A72 (10, -43.7058) -> (9.8, -43.5058) centre (9.8, -43.7058) ccw
  line L75 (10, -48.5058) -> (10, -43.7058)
  arc A73 (8.5, -50.0058) -> (10, -48.5058) centre (8.5, -48.5058) ccw
  line L76 (3.75, -50.0058) -> (8.5, -50.0058)
  arc A74 (3.55, -49.8058) -> (3.75, -50.0058) centre (3.75, -49.8058) ccw
  line L77 (3.55, -49.7058) -> (3.55, -49.8058)
  arc A75 (3.55, -49.7058) -> (3.35, -49.5058) centre (3.35, -49.7058) ccw
  line L78 (3.2, -49.5058) -> (3.35, -49.5058)
  arc A76 (3, -49.3058) -> (3.2, -49.5058) centre (3.2, -49.3058) ccw
  line L79 (3, -49.0058) -> (3, -49.3058)
  arc A77 (3.5, -48.5058) -> (3, -49.0058) centre (3.5, -49.0058) ccw
  line L80 (5.5, -48.5058) -> (3.5, -48.5058)
  arc A78 (5.5, -48.5058) -> (6, -48.0058) centre (5.5, -48.0058) ccw
  line L81 (6, -47.2735) -> (6, -48.0058)
  arc A79 (6, -47.2735) -> (5.8536, -46.92) centre (5.5, -47.2735) ccw
  line L82 (3.5858, -44.6522) -> (5.8536, -46.92)
  arc A80 (3.5858, -44.6522) -> (3.2322, -44.5058) centre (3.2322, -45.0058) ccw
  line L83 (0.9536, -44.5058) -> (3.2322, -44.5058)
  arc A81 (0.8536, -44.479) -> (0.9536, -44.5058) centre (0.9536, -44.3058) ccw
  line L84 (0.1, -44.0439) -> (0.8536, -44.479)
  arc A82 (0.1, -44.0439) -> (-0.1, -44.0439) centre (0, -44.2171) ccw
  line L85 (-0.8536, -44.479) -> (-0.1, -44.0439)
  arc A83 (-0.9536, -44.5058) -> (-0.8536, -44.479) centre (-0.9536, -44.3058) ccw
  line L86 (-3.2322, -44.5058) -> (-0.9536, -44.5058)
  arc A84 (-3.2322, -44.5058) -> (-3.5858, -44.6522) centre (-3.2322, -45.0058) ccw
  line L87 (-5.8536, -46.92) -> (-3.5858, -44.6522)
  arc A85 (-5.8536, -46.92) -> (-6, -47.2735) centre (-5.5, -47.2735) ccw
  arc A86 (-3.5858, -35.3593) -> (-3.2322, -35.5058) centre (-3.2322, -35.0058) ccw
  line L88 (-3.2322, -35.5058) -> (-0.9536, -35.5058)
  arc A87 (-0.8536, -35.5326) -> (-0.9536, -35.5058) centre (-0.9536, -35.7058) ccw
  line L89 (-0.8536, -35.5326) -> (-0.1, -35.9677)
  arc A88 (-0.1, -35.9677) -> (0.1, -35.9677) centre (0, -35.7945) ccw
  line L90 (0.1, -35.9677) -> (0.8536, -35.5326)
  arc A89 (0.9536, -35.5058) -> (0.8536, -35.5326) centre (0.9536, -35.7058) ccw
  line L91 (0.9536, -35.5058) -> (3.2322, -35.5058)
  arc A90 (3.2322, -35.5058) -> (3.5858, -35.3593) centre (3.2322, -35.0058) ccw
  line L92 (3.5858, -35.3593) -> (8.5, -30.4451)
  line L93 (8.5, -30.4451) -> (8.5, -9.5607)
  line L94 (8.5, -9.5607) -> (3.5858, -4.6464)
  arc A91 (3.5858, -4.6464) -> (3.2322, -4.5) centre (3.2322, -5) ccw
  line L95 (3.2322, -4.5) -> (0.9536, -4.5)
  arc A92 (0.8536, -4.4732) -> (0.9536, -4.5) centre (0.9536, -4.3) ccw
  line L96 (0.8536, -4.4732) -> (0.1, -4.0381)
  arc A93 (0.1, -4.0381) -> (-0.1, -4.0381) centre (0, -4.2113) ccw
  line L97 (-0.1, -4.0381) -> (-0.8536, -4.4732)
  arc A94 (-0.9536, -4.5) -> (-0.8536, -4.4732) centre (-0.9536, -4.3) ccw
  line L98 (-0.9536, -4.5) -> (-3.2322, -4.5)
  arc A95 (-3.2322, -4.5) -> (-3.5858, -4.6464) centre (-3.2322, -5) ccw
  line L99 (-3.5858, -4.6464) -> (-8.5, -9.5607)
  line L100 (-8.5, -9.5607) -> (-8.5, -30.4451)
  arc A96 (-9.8, -3.55) -> (-10, -3.75) centre (-9.8, -3.75) ccw
  line L101 (-9.7, -3.55) -> (-9.8, -3.55)
  arc A97 (-9.7, -3.55) -> (-9.5, -3.35) centre (-9.7, -3.35) ccw
  line L102 (-9.5, -3.25) -> (-9.5, -3.35)
  arc A98 (-9.3, -3.05) -> (-9.5, -3.25) centre (-9.3, -3.25) ccw
  line L103 (-9, -3.05) -> (-9.3, -3.05)
  arc A99 (-8.5, -3.55) -> (-9, -3.05) centre (-9, -3.55) ccw
  line L104 (-8.5, -5.5) -> (-8.5, -3.55)
  arc A100 (-8.5, -5.5) -> (-8, -6) centre (-8, -5.5) ccw
  line L105 (-7.2678, -6) -> (-8, -6)
  arc A101 (-7.2678, -6) -> (-6.9142, -5.8536) centre (-7.2678, -5.5) ccw
  line L106 (-4.7214, -3.6608) -> (-6.9142, -5.8536)
  arc A102 (-4.7214, -3.6608) -> (-4.575, -3.3072) centre (-5.075, -3.3072) ccw
  line L107 (-4.575, -0.8286) -> (-4.575, -3.3072)
  arc A103 (-4.5482, -0.7286) -> (-4.575, -0.8286) centre (-4.375, -0.8286) ccw
  line L108 (-4.142, -0.025) -> (-4.5482, -0.7286)
  arc A104 (-4.142, -0.025) -> (-4.142, 0.175) centre (-4.3152, 0.075) ccw
  line L109 (-4.5482, 0.8786) -> (-4.142, 0.175)
  arc A105 (-4.575, 0.9786) -> (-4.5482, 0.8786) centre (-4.375, 0.9786) ccw
  line L110 (-4.575, 3.3072) -> (-4.575, 0.9786)
  arc A106 (-4.575, 3.3072) -> (-4.7214, 3.6608) centre (-5.075, 3.3072) ccw
  line L111 (-6.9142, 5.8536) -> (-4.7214, 3.6608)
  arc A107 (-6.9142, 5.8536) -> (-7.2678, 6) centre (-7.2678, 5.5) ccw
  line L112 (-8, 6) -> (-7.2678, 6)
  arc A108 (-8, 6) -> (-8.5, 5.5) centre (-8, 5.5) ccw
  line L113 (-8.5, 3.45) -> (-8.5, 5.5)
  arc A109 (-9, 2.95) -> (-8.5, 3.45) centre (-9, 3.45) ccw
  line L114 (-9.3, 2.95) -> (-9, 2.95)
  arc A110 (-9.5, 3.15) -> (-9.3, 2.95) centre (-9.3, 3.15) ccw
  line L115 (-9.5, 3.25) -> (-9.5, 3.15)
  arc A111 (-9.5, 3.25) -> (-9.7, 3.45) centre (-9.7, 3.25) ccw
  line L116 (-9.8, 3.45) -> (-9.7, 3.45)
  arc A112 (-10, 3.65) -> (-9.8, 3.45) centre (-9.8, 3.65) ccw
  line L117 (-10, 8.4942) -> (-10, 3.65)
  arc A113 (-8.5, 9.9942) -> (-10, 8.4942) centre (-8.5, 8.4942) ccw
  line L118 (-3.75, 9.9942) -> (-8.5, 9.9942)
  arc A114 (-3.55, 9.7942) -> (-3.75, 9.9942) centre (-3.75, 9.7942) ccw
  line L119 (-3.55, 9.6942) -> (-3.55, 9.7942)
  arc A115 (-3.55, 9.6942) -> (-3.35, 9.4942) centre (-3.35, 9.6942) ccw
  line L120 (-3.2, 9.4942) -> (-3.35, 9.4942)
  arc A116 (-3, 9.2942) -> (-3.2, 9.4942) centre (-3.2, 9.2942) ccw
  line L121 (-3, 8.9942) -> (-3, 9.2942)
  arc A117 (-3.5, 8.4942) -> (-3, 8.9942) centre (-3.5, 8.9942) ccw
  line L122 (-5.5, 8.4942) -> (-3.5, 8.4942)
  arc A118 (-5.5, 8.4942) -> (-6, 7.9942) centre (-5.5, 7.9942) ccw
  line L123 (-6, 7.262) -> (-6, 7.9942)
  arc A119 (-6, 7.262) -> (-5.8536, 6.9084) centre (-5.5, 7.262) ccw
  line L124 (-3.5858, 4.6407) -> (-5.8536, 6.9084)
  arc A120 (-3.5858, 4.6407) -> (-3.2322, 4.4942) centre (-3.2322, 4.9942) ccw
  line L125 (-0.9536, 4.4942) -> (-3.2322, 4.4942)
  arc A121 (-0.8536, 4.4674) -> (-0.9536, 4.4942) centre (-0.9536, 4.2942) ccw
  line L126 (-0.0592, 4.0088) -> (-0.8536, 4.4674)
  arc A122 (-0.0592, 4.0088) -> (0.0592, 4.0088) centre (0, 4.1113) ccw
  line L127 (0.8536, 4.4674) -> (0.0592, 4.0088)
  arc A123 (0.9536, 4.4942) -> (0.8536, 4.4674) centre (0.9536, 4.2942) ccw
  line L128 (3.2322, 4.4942) -> (0.9536, 4.4942)
  arc A124 (3.2322, 4.4942) -> (3.5858, 4.6407) centre (3.2322, 4.9942) ccw
  line L129 (5.8536, 6.9084) -> (3.5858, 4.6407)
  arc A125 (5.8536, 6.9084) -> (6, 7.262) centre (5.5, 7.262) ccw
  line L130 (6, 7.9942) -> (6, 7.262)
  arc A126 (6, 7.9942) -> (5.5, 8.4942) centre (5.5, 7.9942) ccw
  line L131 (3.5, 8.4942) -> (5.5, 8.4942)
  arc A127 (3, 8.9942) -> (3.5, 8.4942) centre (3.5, 8.9942) ccw
  line L132 (3, 9.2942) -> (3, 8.9942)
  arc A128 (3.2, 9.4942) -> (3, 9.2942) centre (3.2, 9.2942) ccw
  line L133 (3.35, 9.4942) -> (3.2, 9.4942)
  arc A129 (3.35, 9.4942) -> (3.55, 9.6942) centre (3.35, 9.6942) ccw
  line L134 (3.55, 9.7942) -> (3.55, 9.6942)
  arc A130 (3.75, 9.9942) -> (3.55, 9.7942) centre (3.75, 9.7942) ccw
  line L135 (8.5, 9.9942) -> (3.75, 9.9942)
  arc A131 (10, 8.4942) -> (8.5, 9.9942) centre (8.5, 8.4942) ccw
  constraints: 1 other
extrude "Extrusion3" add sketch "Sketch1" along normal blind 20
body "Solid2"
